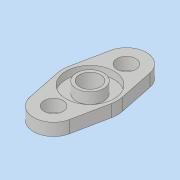
# Autodesk Inventor part: tetherSeal
Saved by Autodesk Inventor 2017.3 (Build 213256000, 256)
## iProperties
Created: 2018-09-08
Part Number: tetherSeal
Material: Generic
Document SubType Name: Modeling
Designer: Derek Wider
Density: 1 g/cm^3
Appearance: Default
Author: Derek Wider
Autodesk Inventor part; units mm, degrees
ref_plane "YZ Plane" through (0, 0, 0) normal (1, 0, 0) x (0, 1, 0)
ref_plane "XZ Plane" through (0, 0, 0) normal (0, 1, 0) x (-1, 0, 0)
ref_plane "XY Plane" through (0, 0, 0) normal (0, 0, 1) x (1, 0, 0)
sketch "Sketch1" plane through (0, 0, 0) normal (0, 1, 0) x (-1, 0, 0)
  circle A0 centre (0, 0) radius 1.8415
  circle A1 centre (0, 0) radius 2.3813
  circle A2 centre (0, -6.35) radius 1.651
  circle A3 centre (0, 6.35) radius 1.651
  arc A4 (3.4219, 7.0485) -> (-3.4219, 7.0485) centre (0, 6.35) ccw
  arc A5 (-3.4219, -7.0485) -> (3.4219, -7.0485) centre (0, -6.35) ccw
  line L0 (3.4219, 7.0485) -> (4.6663, 0.9525)
  line L1 (-3.4219, 7.0485) -> (-4.6663, 0.9525)
  line L2 (3.4219, -7.0485) -> (4.6663, -0.9525)
  line L3 (-3.4219, -7.0485) -> (-4.6663, -0.9525)
  arc A6 (4.6663, -0.9525) -> (4.6663, 0.9525) centre (0, 0) ccw
  arc A7 (-4.6663, 0.9525) -> (-4.6663, -0.9525) centre (0, 0) ccw
  dimension "d0" = 3.683
  dimension "d1" = 4.7625
  dimension "d3" = 3.302
  dimension "d4" = 3.302
  dimension "d5" = 6.985
  dimension "d6" = 6.985
  dimension "d7" = 6.35
  dimension "d8" = 6.35
  dimension "d9" = 4.7625
  constraints: 8 centre point, 8 end point, 8 point on circle, 8 tangent, 5 coincident, 2 vertical alignment, 1 concentric
  measures "d0" diameter of A0
  measures "d1" diameter of A1
  measures "d3" diameter of A2
  measures "d4" diameter of A3
  measures "d5" diameter of A4
  measures "d6" diameter of A5
  measures "d7" distance of A3.centre point (0, 0)
  measures "d8" distance of point (0, 0) A2.centre
  measures "d9" radius of A6
extrude "Extrusion1" add sketch "Sketch1" along normal blind 2.159 contours A1 | L0 A6 L2 A5 L3 A7 L1 A4
extrude "Extrusion2" add sketch "Sketch1" along normal blind 2.794 contours A1
sketch "Sketch3" plane through (0, 2.159, 0) normal (0, 1, 0) x (1, 0, 0)
  circle A0 centre (0, 0) radius 4.191
  circle A1 centre (0, 0) radius 2.3813 projected
  dimension "d14" = 8.382
  constraints: 1 centre point, 1 coincident
  measures "d14" diameter of A0
extrude "Extrusion3" cut sketch "Sketch3" against normal blind 1.27
equation "\"d8\" = d7"
body "Solid1"
